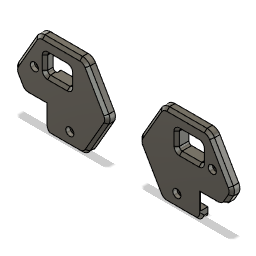
Z Belt Covers (Autodesk Fusion 360 design; units mm, degrees)
Autodesk Fusion 360 part; units mm, degrees
note: some values were not read from the file. Set by a fixed rule: which sketch regions a step uses.
imported_body "Base Feature1" makes body 1
sketch "Sketch1" plane through (0, 0, -38.096) normal (0, 0, -1) x (-1, 0, 0)
  arc A0 (59.4414, 11.0001) -> (57.4414, 13.0001) centre (57.4414, 11.0001) ccw
  line L0 (59.4414, 11.0001) -> (59.4414, 8.6001)
  arc A1 (59.4414, 8.6001) -> (60.4414, 7.6001) centre (60.4414, 8.6001) ccw
  line L1 (60.4414, 7.6001) -> (77, 7.6001)
  arc A2 (77, 7.6001) -> (78, 8.6001) centre (77, 8.6001) ccw
  line L2 (78, 8.6001) -> (78, 18.0004)
  arc A3 (78, 18.0004) -> (73, 23.0004) centre (73, 18.0004) ccw
  line L3 (73, 23.0004) -> (37.9599, 23.0004)
  arc A4 (37.9599, 23.0004) -> (32.9599, 18.0004) centre (37.9599, 18.0004) ccw
  line L4 (32.9599, 18.0004) -> (32.9599, -32.9999)
  arc A5 (32.9599, -32.9999) -> (37.9599, -37.9999) centre (37.9599, -32.9999) ccw
  line L5 (37.9599, -37.9999) -> (55.9999, -37.9999)
  arc A6 (55.9999, -37.9999) -> (57.9999, -35.9999) centre (55.9999, -35.9999) ccw
  line L6 (57.9999, -35.9999) -> (57.9999, -18.8)
  arc A7 (58.7999, -18) -> (57.9999, -18.8) centre (58.7999, -18.8) ccw
  line L7 (58.7999, -18) -> (76, -18)
  arc A8 (76, -18) -> (78, -16) centre (76, -16) ccw
  line L8 (78, -16) -> (78, 3.6001)
  arc A9 (78, 3.6001) -> (77, 4.6001) centre (77, 3.6001) ccw
  line L9 (77, 4.6001) -> (60.4414, 4.6001)
  arc A10 (60.4414, 4.6001) -> (59.4414, 3.6001) centre (60.4414, 3.6001) ccw
  line L10 (59.4414, 3.6001) -> (59.4414, 1.2001)
  arc A11 (57.4414, -0.7999) -> (59.4414, 1.2001) centre (57.4414, 1.2001) ccw
  line L11 (57.4414, -0.7999) -> (44.9595, -0.7999)
  arc A12 (42.9595, 1.2001) -> (44.9595, -0.7999) centre (44.9595, 1.2001) ccw
  line L12 (42.9595, 1.2001) -> (42.9595, 11.0001)
  arc A13 (44.9595, 13.0001) -> (42.9595, 11.0001) centre (44.9595, 11.0001) ccw
  line L13 (44.9595, 13.0001) -> (57.4414, 13.0001)
  circle A14 centre (47.9999, -27.9999) radius 1.7
  line L14 (57.9999, -18) -> (97.9999, -18)
  line L15 (97.9999, -18) -> (97.9999, -58)
  line L16 (97.9999, -58) -> (57.9999, -58)
  line L17 (57.9999, -58) -> (57.9999, -18)
  line L18 (57.9999, -18) -> (77.9999, -18)
  line L19 (77.9999, 23) -> (57.9999, 23)
  line L20 (57.9999, 23) -> (32.9599, 23)
  line L21 (32.9599, 23) -> (32.9599, -37.9999)
  line L22 (32.9599, -37.9999) -> (57.9999, -37.9999)
  line L23 (57.9999, 23) -> (57.9999, 12.9205)
  line L24 (57.9999, -0.7204) -> (57.9999, -18)
  line L25 (57.9999, -37.9999) -> (57.9999, -0.7204)
  line L26 (57.9999, 12.9205) -> (57.9999, 23)
  line L27 (77.9999, -18) -> (77.9999, 3.6123)
  line L28 (77.9999, 8.5879) -> (77.9999, 23)
  line L29 (42.9595, 13.0001) -> (59.4414, 13.0001)
  line L30 (59.4414, 13.0001) -> (59.4414, -0.7999)
  line L31 (59.4414, -0.7999) -> (42.9595, -0.7999)
  line L32 (42.9595, -0.7999) -> (42.9595, 13.0001)
  line L33 (78, 8.6001) -> (77.9999, 3.6123)
  line L34 (77.9999, 4.6001) -> (77.9999, 7.6001)
  line L35 (77.9999, 7.6001) -> (59.4414, 7.6001)
  line L36 (59.4414, 7.6001) -> (59.4414, 4.6001)
  line L37 (59.4414, 4.6001) -> (77.9999, 4.6001)
  circle A15 centre (42.9999, -27.9999) radius 1.7
  line L38 (32.9599, -37.9999) -> (32.9599, 23)
  line L39 (32.9599, 23) -> (27.9599, 23)
  line L40 (27.9599, 23) -> (27.9599, -37.9999)
  line L41 (27.9599, -37.9999) -> (32.9599, -37.9999)
  line L42 (42.9595, 13.0001) -> (42.9595, -0.7999)
  line L43 (42.9595, -0.7999) -> (40.9595, -0.7999)
  line L44 (40.9595, -0.7999) -> (40.9595, 13.0001)
  line L45 (40.9595, 13.0001) -> (42.9595, 13.0001)
  dimension "d1" = 40
  dimension "d2" = 40
  dimension "d3" = 20
  dimension "d4" = 41
  dimension "d5" = 5
  dimension "d81" = 2
  constraint horizontal L14
  constraint vertical L15
  constraint horizontal L16
  constraint vertical L17
  constraint collinear L7 L14
  constraint collinear L6 L17
  constraint horizontal L18
  constraint vertical L27
  constraint horizontal L19
  constraint vertical L23
  constraint horizontal L20
  constraint vertical L21
  constraint horizontal L22
  constraint vertical L25
  constraint coincident A0 L23.end
  constraint coincident A11 L24.start
  constraint collinear L23 L24
  constraint collinear L25 L26
  constraint coincident A9 L27.end
  constraint coincident A2 L28.start
  constraint collinear L27 L28
  constraint horizontal L29
  constraint vertical L30
  constraint horizontal L31
  constraint vertical L32
  constraint collinear L11 L31
  constraint collinear L13 L29
  constraint coincident A2.end L2.start
  constraint perpendicular L34 L35
  constraint parallel L34 L36
  constraint parallel L35 L37
  constraint perpendicular L1 L34
  constraint coincident L33 L34.start
  constraint perpendicular L38 L39
  constraint parallel L38 L40
  constraint parallel L39 L41
  constraint perpendicular L42 L43
  constraint parallel L42 L44
  constraint parallel L43 L45
  measures "d1" distance of L14.start L14.end
  measures "d2" distance of L14.start L16.end
  measures "d3" distance of L14.start L18.end
  measures "d4" distance of L14.start L19.end
  measures "d5" distance of L21.end L40.end
  measures "d81" distance of L29.start L44.end
extrude "Extrude1" add sketch "Sketch1" against normal blind 6 separate body contours L0 A1 L1 A2 L2 A3 L3 L19 L23 L26 L28 L29 L30 L33 L35 | A1 L30 L35 | L3 A4 L4 A5 L5 A6 L6 L11 L13 L17 L20 L21 L22 L23 L24 L25 L26 L29 L31 L38 L43 L44 L45 | L1 L9 L30 L33 L34 L35 L36 L37 | A2 L33 L35 | A10 L30 L37 | A3 L19 L28 | A4 L20 L21 L38 | L7 A8 L8 A9 L9 A10 L10 L14 L18 L24 L25 L27 L30 L31 L37 | L4 L21 L38 L39 L40 L41 | A9 L33 L37 | A5 L21 L22 L38 | A6 L17 L22 L25 | A8 L14 L18 L27 | A14 | A15 makes body 2
extrude "Extrude2" cut 1 faces at (-78, 6.6001, -36.096) along direction (-1, 0, 0) blind 4 on bodies 2 bodies 2
sketch "Sketch2" plane through (0, 0, -32.096) normal (0, 0, 1) x (1, 0, 0)
  line L0 (-78, 7.6001) -> (-77.9999, 7.6001)
  line L1 (-59.4414, 13.0001) -> (-40.9595, 13.0001)
  line L2 (-40.9595, -0.7999) -> (-59.4414, -0.7999)
  line L3 (-59.4414, -0.7999) -> (-59.4414, 13.0001)
  line L4 (-77.9999, 4.6001) -> (-77.9999, 3.6123)
  line L5 (-77.9999, 3.6123) -> (-77.9999, -18)
  line L6 (-77.9999, -18) -> (-57.9999, -18)
  line L7 (-57.9999, -18) -> (-57.9999, -37.9999)
  line L8 (-57.9999, -37.9999) -> (-27.9599, -37.9999)
  line L9 (-27.9599, -37.9999) -> (-27.9599, 23)
  line L10 (-27.9599, 23) -> (-77.9999, 23)
  line L11 (-77.9999, 23) -> (-77.9999, 8.5879)
  arc A0 (-78, 8.6001) -> (-77.9999, 8.5879) centre (-77, 8.6001) ccw
  line L12 (-57.9999, -18) -> (-97.9999, -18) construction
  line L13 (-97.9999, -18) -> (-97.9999, -58) construction
  line L14 (-97.9999, -58) -> (-57.9999, -58) construction
  line L15 (-57.9999, -58) -> (-57.9999, -18) construction
  line L16 (-77.9999, 7.6001) -> (-77.9999, 4.6001)
  line L17 (-78, 8.6001) -> (-78, 7.6001)
  line L18 (-40.9595, 13.0001) -> (-40.9595, -0.7999)
  dimension "d10" = 40
  dimension "d11" = 40
  constraint horizontal L12
  constraint vertical L13
  constraint horizontal L14
  constraint vertical L15
  constraint coincident L6.end L7.start
  measures "d10" distance of L6.end L12.end
  measures "d11" distance of L6.end L14.end
sketch "Sketch3" plane through (0, 0, -32.096) normal (0, 0, 1) x (1, 0, 0)
  line L0 (-78, 7.6001) -> (-77.9999, 7.6001)
  line L1 (-59.4414, 13.0001) -> (-40.9595, 13.0001)
  line L2 (-40.9595, -0.7999) -> (-59.4414, -0.7999)
  line L3 (-59.4414, -0.7999) -> (-59.4414, 13.0001)
  line L4 (-77.9999, 4.6001) -> (-77.9999, 3.6123)
  line L5 (-77.9999, 3.6123) -> (-77.9999, -18)
  line L6 (-77.9999, -18) -> (-57.9999, -18)
  line L7 (-57.9999, -18) -> (-57.9999, -37.9999)
  line L8 (-57.9999, -37.9999) -> (-27.9599, -37.9999)
  line L9 (-27.9599, -37.9999) -> (-27.9599, 23)
  line L10 (-27.9599, 23) -> (-77.9999, 23)
  line L11 (-77.9999, 23) -> (-77.9999, 8.5879)
  arc A0 (-78, 8.6001) -> (-77.9999, 8.5879) centre (-77, 8.6001) ccw
  line L12 (-57.9999, -37.9999) -> (-27.9599, -37.9999) construction
  line L13 (-27.9599, -37.9999) -> (-27.9599, -17.9999) construction
  line L14 (-27.9599, -17.9999) -> (-57.9999, -17.9999) construction
  line L15 (-57.9999, -17.9999) -> (-57.9999, -37.9999) construction
  line L16 (-57.9999, -18) -> (-77.9999, -18) construction
  line L17 (-77.9999, -18) -> (-77.9999, 23) construction
  line L18 (-77.9999, 23) -> (-57.9999, 23) construction
  line L19 (-57.9999, 23) -> (-57.9999, -18) construction
  line L20 (-63.9999, -30.9999) -> (-57.9999, -30.9999) construction
  line L21 (-57.9999, -30.9999) -> (-57.9999, -24.9999) construction
  line L22 (-57.9999, -24.9999) -> (-63.9999, -24.9999) construction
  line L23 (-63.9999, -24.9999) -> (-63.9999, -30.9999) construction
  line L24 (-57.9999, -30.9999) -> (-49.9999, -30.9999)
  line L25 (-49.9999, -30.9999) -> (-49.9999, -7.9999)
  line L26 (-49.9999, -7.9999) -> (-57.9999, -7.9999)
  line L27 (-57.9999, -7.9999) -> (-57.9999, -30.9999)
  line L28 (-61.254, -34.254) -> (-46.7458, -34.254)
  line L29 (-46.7458, -34.254) -> (-46.7458, -4.7458)
  line L30 (-46.7458, -4.7458) -> (-61.254, -4.7458)
  line L31 (-61.254, -4.7458) -> (-61.254, -34.254)
  line L32 (-77.9999, 7.6001) -> (-77.9999, 4.6001)
  line L33 (-78, 8.6001) -> (-78, 7.6001)
  line L34 (-40.9595, 13.0001) -> (-40.9595, -0.7999)
  dimension "d12" = 20
  dimension "d13" = 6
  dimension "d14" = 6
  dimension "d15" = 8
  dimension "d16" = 23
  dimension "d19" = 3.2541
  constraint horizontal L12
  constraint vertical L13
  constraint horizontal L14
  constraint vertical L15
  constraint coincident L9 L13.end
  constraint coincident L7.end L8.start
  constraint horizontal L16
  constraint vertical L17
  constraint horizontal L18
  constraint vertical L19
  constraint coincident L10 L11.start
  constraint coincident L11 L10.end
  constraint coincident L6.end L7.start
  constraint horizontal L20
  constraint vertical L21
  constraint horizontal L22
  constraint vertical L23
  constraint midpoint L15 L21
  constraint horizontal L24
  constraint vertical L25
  constraint horizontal L26
  constraint vertical L27
  measures "d12" distance of L7.end L14.end
  measures "d13" distance of L20.start L20.end
  measures "d14" distance of L20.start L22.end
  measures "d15" distance of L20.end L24.end
  measures "d16" distance of L20.end L26.end
extrude "Extrude3" cut sketch "Sketch3" against normal blind 6 contours L7 L24 L25 L26 L27 bodies 2
extrude "Extrude4" add sketch "Sketch3" against normal blind 1.5 contours L7 L24 L25 L26 L27 bodies 2
extrude "Extrude5" cut 1 faces at (-27.9599, 2.6667, -36.096) along direction (-1, 0, 0) blind 0.04 on bodies 2 bodies 2
extrude "Extrude6" add 1 faces at (-27.9999, 2.6667, -36.096) along direction (1, 0, 0) blind 11 on bodies 2 bodies 2
sketch "Sketch4" plane through (0, 0, -32.096) normal (0, 0, 1) x (1, 0, 0)
  line L0 (-16.9999, 23) -> (-77.9999, 23)
  line L1 (-77.9999, 23) -> (-77.9999, 8.5879)
  arc A0 (-78, 8.6001) -> (-77.9999, 8.5879) centre (-77, 8.6001) ccw
  line L2 (-78, 8.6001) -> (-78, 7.6001)
  line L3 (-78, 7.6001) -> (-77.9999, 7.6001)
  line L4 (-77.9999, 7.6001) -> (-77.9999, 4.6001)
  line L5 (-77.9999, 4.6001) -> (-77.9999, 3.6123)
  line L6 (-77.9999, 3.6123) -> (-77.9999, -18)
  line L7 (-77.9999, -18) -> (-57.9999, -18)
  line L8 (-57.9999, -18) -> (-57.9999, -37.9999)
  line L9 (-57.9999, -37.9999) -> (-16.9999, -37.9999)
  line L10 (-16.9999, -37.9999) -> (-16.9999, 23)
  line L11 (-59.4414, -0.7999) -> (-59.4414, 13.0001)
  line L12 (-59.4414, 13.0001) -> (-40.9595, 13.0001)
  line L13 (-40.9595, -0.7999) -> (-59.4414, -0.7999)
  line L14 (-77.9999, 23) -> (-16.9999, -37.9999) construction
  line L15 (-65.1091, 23) -> (-82.7182, -7.5)
  line L16 (-82.7182, -7.5) -> (-65.1091, -37.9999)
  line L17 (-65.1091, -37.9999) -> (-29.8908, -37.9999)
  line L18 (-29.8908, -37.9999) -> (-12.2816, -7.5)
  line L19 (-12.2816, -7.5) -> (-29.8908, 23)
  line L20 (-29.8908, 23) -> (-65.1091, 23)
  line L21 (-40.9595, 13.0001) -> (-40.9595, -0.7999)
  point P0 (-47.4999, -7.5)
  dimension "d27" = 30.5
  constraint coincident L0.end L1.start
  constraint coincident L9.end L10.start
  constraint midpoint L14 P0
  measures "d27" distance of P0 L20
extrude "Extrude7" add sketch "Sketch4" against normal blind 6 contours L10 L18 L19 | L6 L15 L16 bodies 2
extrude "Extrude8" cut sketch "Sketch4" against normal blind 6 contours L0 L10 L19 | L0 L1 A0 L2 L4 L5 L6 L15 | L9 L10 L18 | L6 L7 L16 bodies 2
sketch "Sketch5" plane through (0, 0, -32.096) normal (0, 0, 1) x (1, 0, 0)
  line L0 (-12.2816, -7.5) -> (-29.8908, 23)
  line L1 (-29.8908, 23) -> (-65.1091, 23)
  line L2 (-65.1091, 23) -> (-82.7182, -7.5)
  line L3 (-82.7182, -7.5) -> (-76.656, -18)
  line L4 (-76.656, -18) -> (-57.9999, -18)
  line L5 (-57.9999, -18) -> (-57.9999, -37.9999)
  line L6 (-57.9999, -37.9999) -> (-29.8908, -37.9999)
  line L7 (-29.8908, -37.9999) -> (-12.2816, -7.5)
  line L8 (-59.4414, -0.7999) -> (-59.4414, 13.0001)
  line L9 (-59.4414, 13.0001) -> (-40.9595, 13.0001)
  line L10 (-40.9595, -0.7999) -> (-59.4414, -0.7999)
  line L11 (-57.9999, -28) -> (-24.1173, -28) construction
  line L12 (-67.328, -18) -> (-67.328, 19.1568) construction
  circle A0 centre (-41.0586, -28) radius 1.7
  circle A1 centre (-67.328, 0.5784) radius 1.7
  line L13 (-40.9595, 13.0001) -> (-40.9595, -0.7999)
  dimension "d54" = 90
  dimension "d55" = 3.4
  dimension "d56" = 3.4
  constraint midpoint L5 L11.start
  constraint coincident L7 L11.end
  constraint perpendicular L5 L11
  constraint midpoint L4 L12.start
  constraint coincident L2 L12.end
  constraint midpoint L11 A0.centre
  constraint midpoint L12 A1.centre
  measures "d54" angle of L11 L12
  measures "d55" diameter of A0
  measures "d56" diameter of A1
extrude "Extrude9" cut sketch "Sketch5" against normal blind 6 contours A0 | A1 bodies 2
fillet "Fillet1" radius 2.5 1 edges at (-57.9999, -18, -35.846) on bodies 2
fillet "Fillet2" radius 1.5 3 edges at (-49.9999, -30.9999, -35.846) (-49.9999, -7.9999, -35.846) (-57.9999, -7.9999, -35.846) on bodies 2
fillet "Fillet3" radius 6.5 5 edges at (-12.2816, -7.5, -35.096) (-29.8908, -37.9999, -35.096) (-29.8908, 23, -35.096) (-65.1091, 23, -35.096) (-82.7182, -7.5, -35.096) on bodies 2
chamfer "Chamfer2" distance 2 angle 45 11 edges at (-21.0862, -22.7499, -32.096) (-13.2871, -7.5, -32.096) (-21.0862, 7.75, -32.096) (-30.3935, 22.1292, -32.096) (-47.4999, 23, -32.096) (-64.6063, 22.1292, -32.096) (-73.9137, 7.75, -32.096) (-81.7127, -7.5, -32.096) (-78.7489, -14.375, -32.096) (-45.8217, -37.9999, -32.096) (-30.3935, -37.1291, -32.096) on bodies 2
sketch "Sketch9" plane through (0, 0, -32.096) normal (0, 0, 1) x (1, 0, 0)
  line L0 (-79.1098, -9.75) -> (-74.3466, -18)
  line L1 (-74.3466, -18) -> (-57.9999, -18)
  line L2 (-57.9999, -18) -> (-57.9999, -35.9999)
  line L3 (-57.9999, -35.9999) -> (-33.6435, -35.9999)
  arc A0 (-33.6435, -35.9999) -> (-29.7464, -33.7499) centre (-33.6435, -31.4999) ccw
  line L4 (-29.7464, -33.7499) -> (-15.89, -9.75)
  arc A1 (-15.89, -9.75) -> (-15.89, -5.25) centre (-19.7871, -7.5) ccw
  line L5 (-15.89, -5.25) -> (-29.7464, 18.75)
  arc A2 (-29.7464, 18.75) -> (-33.6435, 21) centre (-33.6435, 16.5) ccw
  line L6 (-33.6435, 21) -> (-61.3563, 21)
  arc A3 (-61.3563, 21) -> (-65.2534, 18.75) centre (-61.3563, 16.5) ccw
  line L7 (-65.2534, 18.75) -> (-79.1098, -5.25)
  arc A4 (-79.1098, -5.25) -> (-79.1098, -9.75) centre (-75.2127, -7.5) ccw
  circle A5 centre (-67.328, 0.5784) radius 1.7
  circle A6 centre (-41.0586, -28) radius 1.7
  line L8 (-59.4414, -0.7999) -> (-59.4414, 13.0001)
  line L9 (-59.4414, 13.0001) -> (-40.9595, 13.0001)
  line L10 (-40.9595, -0.7999) -> (-59.4414, -0.7999)
  line L11 (-63.5214, 17.75) -> (-77.3778, -6.25)
  arc A7 (-77.3778, -6.25) -> (-77.3778, -8.75) centre (-75.2127, -7.5) ccw
  line L12 (-77.3778, -8.75) -> (-73.1919, -16)
  line L13 (-73.1919, -16) -> (-55.9999, -16)
  line L14 (-55.9999, -16) -> (-55.9999, -33.9999)
  line L15 (-55.9999, -33.9999) -> (-33.6435, -33.9999)
  arc A8 (-33.6435, -33.9999) -> (-31.4785, -32.7499) centre (-33.6435, -31.4999) ccw
  line L16 (-31.4785, -32.7499) -> (-17.6221, -8.75)
  arc A9 (-17.6221, -8.75) -> (-17.6221, -6.25) centre (-19.7871, -7.5) ccw
  line L17 (-17.6221, -6.25) -> (-31.4785, 17.75)
  arc A10 (-31.4785, 17.75) -> (-33.6435, 19) centre (-33.6435, 16.5) ccw
  line L18 (-33.6435, 19) -> (-61.3563, 19)
  arc A11 (-61.3563, 19) -> (-63.5214, 17.75) centre (-61.3563, 16.5) ccw
  line L19 (-63.175, 17.55) -> (-77.0313, -6.45)
  arc A12 (-77.0313, -6.45) -> (-77.0313, -8.55) centre (-75.2127, -7.5) ccw
  line L20 (-77.0313, -8.55) -> (-72.961, -15.6)
  line L21 (-72.961, -15.6) -> (-55.5999, -15.6)
  line L22 (-55.5999, -15.6) -> (-55.5999, -33.5999)
  line L23 (-55.5999, -33.5999) -> (-33.6435, -33.5999)
  arc A13 (-33.6435, -33.5999) -> (-31.8249, -32.5499) centre (-33.6435, -31.4999) ccw
  line L24 (-31.8249, -32.5499) -> (-17.9685, -8.55)
  arc A14 (-17.9685, -8.55) -> (-17.9685, -6.45) centre (-19.7871, -7.5) ccw
  line L25 (-17.9685, -6.45) -> (-31.8249, 17.55)
  arc A15 (-31.8249, 17.55) -> (-33.6435, 18.6) centre (-33.6435, 16.5) ccw
  line L26 (-33.6435, 18.6) -> (-61.3563, 18.6)
  arc A16 (-61.3563, 18.6) -> (-63.175, 17.55) centre (-61.3563, 16.5) ccw
  line L27 (-40.9595, 13.0001) -> (-40.9595, -0.7999)
  dimension "d77" = -2
  dimension "d78" = -2.4
sketch "Sketch6" plane through (0, 0, -32.096) normal (0, 0, 1) x (1, 0, 0)
  line L0 (-79.1098, -9.75) -> (-74.3466, -18)
  line L1 (-74.3466, -18) -> (-57.9999, -18)
  line L2 (-57.9999, -18) -> (-57.9999, -35.9999)
  line L3 (-57.9999, -35.9999) -> (-33.6435, -35.9999)
  arc A0 (-33.6435, -35.9999) -> (-29.7464, -33.7499) centre (-33.6435, -31.4999) ccw
  line L4 (-29.7464, -33.7499) -> (-15.89, -9.75)
  arc A1 (-15.89, -9.75) -> (-15.89, -5.25) centre (-19.7871, -7.5) ccw
  line L5 (-15.89, -5.25) -> (-29.7464, 18.75)
  arc A2 (-29.7464, 18.75) -> (-33.6435, 21) centre (-33.6435, 16.5) ccw
  line L6 (-33.6435, 21) -> (-61.3563, 21)
  arc A3 (-61.3563, 21) -> (-65.2534, 18.75) centre (-61.3563, 16.5) ccw
  line L7 (-65.2534, 18.75) -> (-79.1098, -5.25)
  arc A4 (-79.1098, -5.25) -> (-79.1098, -9.75) centre (-75.2127, -7.5) ccw
  circle A5 centre (-41.0586, -28) radius 3
  circle A6 centre (-67.328, 0.5784) radius 3
  circle A7 centre (-67.328, 0.5784) radius 1.7
  circle A8 centre (-41.0586, -28) radius 1.7
  line L8 (-59.4414, -0.7999) -> (-59.4414, 13.0001)
  line L9 (-59.4414, 13.0001) -> (-40.9595, 13.0001)
  line L10 (-40.9595, -0.7999) -> (-59.4414, -0.7999)
  line L11 (-40.9595, 13.0001) -> (-40.9595, -0.7999)
  dimension "d48" = 6
  dimension "d49" = 6
  measures "d48" diameter of A5
  measures "d49" diameter of A6
extrude "Extrude10" cut sketch "Sketch6" against normal blind 3 contours A5 | A6 bodies 2
fillet "Fillet4" radius 3 tangency weight 1.06058 4 edges at (-76.656, -18, -36.096) (-75.5013, -18, -33.096) (-57.9999, -37.9999, -36.096) (-57.9999, -36.9999, -33.096) on bodies 2
fillet "Fillet5" radius 1 1 edges at (-57.9999, -24.5, -33.596) on bodies 2
sketch "Sketch7" plane through (0, 0, -38.096) normal (0, 0, -1) x (-1, 0, 0)
  circle A0 centre (67.328, 0.5784) radius 1.7
  circle A1 centre (41.0586, -28) radius 1.7
  spline S0 degree 3 poles (57.9999, -34.9999) (57.9999, -35.4148) (57.9234, -35.8255) (57.6189, -36.5608) (57.4072, -36.8799) (56.8763, -37.4076) (56.5694, -37.6119) (56.0341, -37.8388) (55.8287, -37.9007) (55.4147, -37.9808) (55.2075, -37.9999) (54.9999, -37.9999) knots 0 0 0 0 0.124473 0.124473 0.239132 0.239132 0.349542 0.349542 0.413866 0.413866 0.476226 0.476226 0.476226 0.476226
  line L0 (57.9999, -34.9999) -> (57.9999, -30.9999)
  line L1 (57.9999, -30.9999) -> (51.4999, -30.9999)
  arc A2 (49.9999, -29.4999) -> (51.4999, -30.9999) centre (51.4999, -29.4999) ccw
  line L2 (49.9999, -29.4999) -> (49.9999, -9.4999)
  arc A3 (51.4999, -7.9999) -> (49.9999, -9.4999) centre (51.4999, -9.4999) ccw
  line L3 (51.4999, -7.9999) -> (56.4999, -7.9999)
  arc A4 (57.9999, -9.4999) -> (56.4999, -7.9999) centre (56.4999, -9.4999) ccw
  line L4 (57.9999, -9.4999) -> (57.9999, -15.5)
  arc A5 (57.9999, -15.5) -> (60.4999, -18) centre (60.4999, -15.5) ccw
  line L5 (60.4999, -18) -> (74.924, -18)
  spline S1 degree 3 poles (77.5221, -16.5) (77.3195, -16.8508) (77.0572, -17.1593) (76.4787, -17.602) (76.1923, -17.7518) (75.5738, -17.9526) (75.2505, -18) (74.924, -18) knots 0 0 0 0 0.121516 0.121516 0.218838 0.218838 0.316843 0.316843 0.316843 0.316843
  line L6 (77.5221, -16.5) -> (80.8419, -10.75)
  arc A6 (80.8419, -10.75) -> (80.8419, -4.25) centre (75.2127, -7.5) ccw
  line L7 (80.8419, -4.25) -> (66.9855, 19.75)
  arc A7 (66.9855, 19.75) -> (61.3563, 23) centre (61.3563, 16.5) ccw
  line L8 (61.3563, 23) -> (33.6435, 23)
  arc A8 (33.6435, 23) -> (28.0144, 19.75) centre (33.6435, 16.5) ccw
  line L9 (28.0144, 19.75) -> (14.158, -4.25)
  arc A9 (14.158, -4.25) -> (14.158, -10.75) centre (19.7871, -7.5) ccw
  line L10 (14.158, -10.75) -> (28.0144, -34.7499)
  arc A10 (28.0144, -34.7499) -> (33.6435, -37.9999) centre (33.6435, -31.4999) ccw
  line L11 (33.6435, -37.9999) -> (54.9999, -37.9999)
  line L12 (59.4414, 13.0001) -> (59.4414, -0.7999)
  line L13 (59.4414, -0.7999) -> (40.9595, -0.7999)
  line L14 (40.9595, 13.0001) -> (59.4414, 13.0001)
  line L15 (57.9999, -30.9999) -> (57.9999, 23)
  line L16 (61.4414, 15.0001) -> (61.4414, -2.7999)
  line L17 (61.4414, -2.7999) -> (40.9595, -2.7999)
  line L18 (40.9595, -2.7999) -> (40.9595, 15.0001)
  line L19 (40.9595, 15.0001) -> (61.4414, 15.0001)
  line L20 (57.4999, -30.9999) -> (57.4999, 23)
  line L21 (40.9595, -0.7999) -> (40.9595, 13.0001)
  line L22 (40.9595, 15.0001) -> (40.9595, -2.7999)
  line L23 (40.9595, -2.7999) -> (38.9595, -2.7999)
  line L24 (38.9595, -2.7999) -> (38.9595, 15.0001)
  line L25 (38.9595, 15.0001) -> (40.9595, 15.0001)
  dimension "d62" = -0.5
  dimension "d82" = 2
  constraint coincident L0.end L1.start
  constraint coincident L8 L15.end
  constraint perpendicular L8 L15
  constraint parallel L12 L16
  constraint parallel L13 L17
  constraint parallel L14 L19
  constraint perpendicular L22 L23
  constraint parallel L22 L24
  constraint parallel L23 L25
  constraint perpendicular L17 L22
  measures "d82" distance of L18.end L24.end
extrude "Extrude11" add sketch "Sketch7" along normal blind 3 contours L13 L17 L18 L20 L22 | L18 L21 L22 L23 L24 L25 | L14 L18 L19 L20 L22 bodies 2
fillet "Fillet6" radius 1 6 edges at (-57.4999, 13.0001, -39.596) (-57.4999, 15.0001, -39.596) (-57.4999, -0.7999, -39.596) (-57.4999, -2.7999, -39.596) (-38.9595, 15.0001, -39.596) (-38.9595, -2.7999, -39.596) on bodies 2
fillet "Fillet7" radius 2 4 edges at (-59.4414, 13.0001, -35.096) (-59.4414, -0.7999, -35.096) (-40.9595, 13.0001, -36.596) (-40.9595, -0.7999, -36.596) on bodies 2
chamfer "Chamfer3" distance 2 angle 45 8 edges at (-50.2005, 13.0001, -32.096) (-41.5453, 12.4143, -32.096) (-40.9595, 6.1001, -32.096) (-41.5453, -0.2141, -32.096) (-50.2005, -0.7999, -32.096) (-58.8557, -0.2141, -32.096) (-59.4414, 6.1001, -32.096) (-58.8557, 12.4143, -32.096) on bodies 2
mirror "Mirror1" about plane through (-59.4414, 7.6001, -38.096) normal (1, 0, 0) of bodies 2 makes body 3
move_body "Move1" bodies 3 to x (1, 0, 0) y (0, 1, 0) z (0, 0, 1) at (116, 0, 0)
hidden bodies 1
